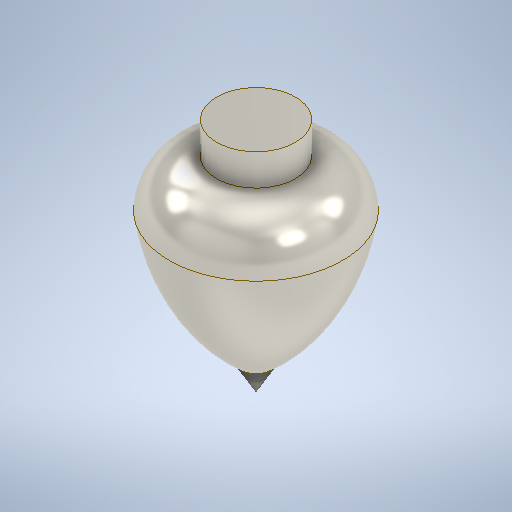
# Autodesk Inventor part: Peao_0001_001
Saved by Autodesk Inventor 2025.2 (Build 292293000, 293)
## iProperties
Created: 2025-03-25
Part Number: Peao_0001_001
Material: Liga de aço
Document SubType Name: Modeling
Designer: lucas
Density: 7.73 g/cm^3
Appearance: Titânio
Author: lucas
Autodesk Inventor part; units mm, degrees
ref_plane "YZ Plane" through (0, 0, 0) normal (1, 0, 0) x (0, 1, 0)
ref_plane "XZ Plane" through (0, 0, 0) normal (0, 1, 0) x (-1, 0, 0)
ref_plane "XY Plane" through (0, 0, 0) normal (0, 0, 1) x (1, 0, 0)
sketch "Esboço1" plane through (0, 0, 0) normal (0, 0, 1) x (1, 0, 0)
  line L0 (-2.5, 5) -> (2.5, 5) construction
  line L1 (-2.5, 5) -> (-2.5, 3)
  line L2 (0, 0) -> (0, -10) construction
  line L3 (0, -10) -> (-1, -8.2679)
  line L4 (-2.5, 5) -> (0, 5)
  line L5 (0, 0) -> (-5.5, 0) construction
  arc A0 (-2.5, 3) -> (-5.5, 0) centre (-2.5, 0) ccw
  line L6 (-2.5, 3) -> (-5.5, 3) construction
  line L7 (-5.5, 3) -> (-5.5, 0) construction
  line L8 (-5.5, 0) -> (-1, -8.2679) construction
  arc A1 (-5.5, 0) -> (-1, -8.2679) centre (7.3937, 1.6591) ccw
  line L9 (0, 5) -> (0, -10)
  line L10 (0, -13) -> (0, 8) projected
  dimension "d0" = 5
  dimension "d1" = 5
  dimension "d2" = 2
  dimension "d3" = 10
  dimension "d4" = 30
  dimension "d5" = 2
  dimension "d7" = 13
  constraints: 20 end point, 4 point on circle, 3 horizontal, 2 centre point, 2 collinear, 2 tangent, 2 vertical, 1 midpoint, 1 perpendicular, 1 vertical alignment
  measures "d0" distance of L0.start L0.end
  measures "d1" distance from line of L2.start L0
  measures "d2" distance of L0.start L1.end
  measures "d3" distance of L2.start L2.end
  measures "d4" angle of L2 L3
  measures "d5" distance of L2.end L3.end
  measures "d7" radius of A1
revolve "Revolução1" add sketch "Esboço1" angle 360 about axis through (0, -10, 0) along (0, 1, 0)
